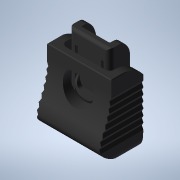
# Autodesk Inventor part: 6321.050_P9 1
Saved by Autodesk Inventor 2021 (Build 250183000, 183)
## iProperties
Created: 2025-05-05
Part Number: 6321.050_P9 1
Material: Generic
Catalog Web Link: www.cadenas.de
Description: AX Bediengehäuse für Tisch-TFT bis 24" - P9-Kompakt-Schaltschränke AX
Vendor: RITTAL
Document SubType Name: Modeling
Designer: psAdmin
Manufacturer: RITTAL
Mass: 3.67605 g
Surface Area: 33.3158 cm^2
Volume: 3.67605 cm^3
Density: 1 g/cm^3
Appearance: PSOLRGB-175-175-175
Category: PARTsolutions
Company: RITTAL
Title: 6321.050_P9 1
Author: Cadenas PARTsolutions
Comments: Kompakt-Schaltschränke AX
PSOL_IDENT_0: {$CADENAS_DATA/23d-libs/rittal/schaltschranksys/kompakt_schaltschr/parts_ae_2_0/bg_ax_fur_tisch_tft_
PSOL_IDENT_1: p9.prj},204 {VTYP=3D},{NB=6321.050_P9 1},{LINA=6321.050_P9 1},{NN=AX Bediengehäuse für Tisch-TFT bis
PSOL_IDENT_2: 24\" - P9},{DATE=28.04.2025 21:11:30},{GEOMDATE=11.04.2025 11:21:47},{VERSION=},{LINEID=40},{WBVAR=
PSOL_IDENT_3: },{WBNUMERIC=}  {NB=6321.050_P9 1},{LINA=6321.050_P9 1},{KT=DUMMY},{BEST=6321.050},{DETAIL=1},{B=650
PSOL_IDENT_4: },{H=450},{VER=1},{GEW=15,8},{CNSETIM80=EC002504},{CNSETIM90=EC002504},{CNSECLASS60=27-18-05-05},{CN
PSOL_IDENT_5: SECLASS80=27-18-05-05},{UNSPSC=31-26-15-02}
NB: 6321.050_P9 1
NN: AX Bediengehäuse für Tisch-TFT bis 24" - P9
NT: Kompakt-Schaltschränke AX
NBSYN: $BEST._P9 $DETAIL.
LINA: 6321.050_P9 1
CATALOG: Rittal
BEST: 6321.050
DETAIL: 1
B: 650
H: 450
VER: 1
GEW: 15,8
CNSETIM80: EC002504
CNSETIM90: EC002504
CNSECLASS60: 27-18-05-05
CNSECLASS80: 27-18-05-05
UNSPSC: 31-26-15-02
SUPPLIER: RITTAL
ARTICLENO: 6321.050_P9 1
BOMINFO: 6321.050_P9 1
CREATOR: CADENAS GmbH
Autodesk Inventor part; units mm, degrees
sketch "Sketch_1" plane through (0, 0, 0) normal (0, 0, 1) x (1, 0, 0)
  line L0 (-10.45, -19.2) -> (-10.45, -21.5)
  arc A0 (-10.45, -21.5) -> (-7.45, -24.5) centre (-7.45, -21.5) ccw
  line L1 (-7.45, -24.5) -> (-2.3229, -24.5)
  arc A1 (-2.3229, -24.5) -> (-1.6614, -24.25) centre (-2.3229, -23.5) ccw
  arc A2 (-1, -24) -> (-1.6614, -24.25) centre (-1, -25) ccw
  line L2 (-1, -24) -> (1, -24)
  arc A3 (1.6614, -24.25) -> (1, -24) centre (1, -25) ccw
  arc A4 (1.6614, -24.25) -> (2.3229, -24.5) centre (2.3229, -23.5) ccw
  line L3 (2.3229, -24.5) -> (7.45, -24.5)
  arc A5 (7.45, -24.5) -> (10.45, -21.5) centre (7.45, -21.5) ccw
  line L4 (10.45, -21.5) -> (10.45, -19.2)
  line L5 (10.45, -19.2) -> (9.95, -18.2)
  line L6 (9.95, -18.2) -> (10.45, -17.2)
  line L7 (10.45, -17.2) -> (9.95, -16.2)
  line L8 (9.95, -16.2) -> (10.45, -15.2)
  line L9 (10.45, -15.2) -> (9.95, -14.2)
  line L10 (9.95, -14.2) -> (10.45, -13.2)
  line L11 (10.45, -13.2) -> (9.95, -12.2)
  line L12 (9.95, -12.2) -> (10.45, -11.2)
  line L13 (10.45, -11.2) -> (9.95, -10.2)
  line L14 (9.95, -10.2) -> (10.45, -9.2)
  line L15 (10.45, -9.2) -> (9.95, -8.2)
  line L16 (9.95, -8.2) -> (10.45, -7.2)
  line L17 (10.45, -7.2) -> (9.95, -6.2)
  line L18 (9.95, -6.2) -> (10.45, -5.2)
  line L19 (10.45, -5.2) -> (10.45, -0.3)
  arc A6 (10.45, -0.3) -> (10.15, 0) centre (10.15, -0.3) ccw
  line L20 (10.15, 0) -> (-10.15, 0)
  arc A7 (-10.15, 0) -> (-10.45, -0.3) centre (-10.15, -0.3) ccw
  line L21 (-10.45, -0.3) -> (-10.45, -5.2)
  line L22 (-10.45, -5.2) -> (-9.95, -6.2)
  line L23 (-9.95, -6.2) -> (-10.45, -7.2)
  line L24 (-10.45, -7.2) -> (-9.95, -8.2)
  line L25 (-9.95, -8.2) -> (-10.45, -9.2)
  line L26 (-10.45, -9.2) -> (-9.95, -10.2)
  line L27 (-9.95, -10.2) -> (-10.45, -11.2)
  line L28 (-10.45, -11.2) -> (-9.95, -12.2)
  line L29 (-9.95, -12.2) -> (-10.45, -13.2)
  line L30 (-10.45, -13.2) -> (-9.95, -14.2)
  line L31 (-9.95, -14.2) -> (-10.45, -15.2)
  line L32 (-10.45, -15.2) -> (-9.95, -16.2)
  line L33 (-9.95, -16.2) -> (-10.45, -17.2)
  line L34 (-10.45, -17.2) -> (-9.95, -18.2)
  line L35 (-9.95, -18.2) -> (-10.45, -19.2)
  constraints: 72 end point, 16 point on circle, 8 centre point
extrude "Extrusion1" add sketch "Sketch_1" along normal blind 14
sketch "Sketch_2" plane through (0, 0, 0) normal (1, 0, 0) x (0, 1, 0)
  line L0 (-28, 20) -> (-28, -5)
  line L1 (-28, -5) -> (5, -5)
  line L2 (5, -5) -> (5, 20)
  line L3 (5, 20) -> (-28, 20)
  arc A0 (-18.0876, 13.9583) -> (-20.637, 12.9256) centre (-18.3613, 10.9708) ccw
  arc A1 (-20.637, 12.9256) -> (-24.5, 2.5) centre (-8.5, 2.5) ccw
  line L4 (-24.5, 2.5) -> (-24.5, 0.5657)
  arc A2 (-24.5, 0.5657) -> (-17, 0) centre (-17, 50) ccw
  line L5 (-17, 0) -> (-4, 0)
  arc A3 (-4, 0) -> (-3.4, 0.2) centre (-4, 1) ccw
  arc A4 (-3.4, 0.2) -> (0, 7) centre (-8.5, 7) ccw
  line L6 (0, 7) -> (0, 10.2)
  arc A5 (0, 10.2) -> (-0.3, 10.5) centre (-0.3, 10.2) ccw
  line L7 (-0.3, 10.5) -> (-3.744, 10.5)
  arc A6 (-14.614, 12.9868) -> (-3.744, 10.5) centre (-3.744, 35.5) ccw
  arc A7 (-14.614, 12.9868) -> (-18.0876, 13.9583) centre (-19, 4) ccw
  constraints: 16 end point, 16 point on circle, 8 centre point
extrude "Extrusion2" cut sketch "Sketch_2" along normal mid plane 22
sketch "Sketch_3" plane through (0, 0, 0) normal (0, 1, 0) x (-1, 0, 0)
  arc A0 (7.95, 1) -> (8.95, 0) centre (8.95, 1) ccw
  line L0 (7.95, 1) -> (7.95, 7)
  arc A1 (7.95, 7) -> (6.45, 8.5) centre (6.45, 7) ccw
  line L1 (6.45, 8.5) -> (-6.45, 8.5)
  arc A2 (-6.45, 8.5) -> (-7.95, 7) centre (-6.45, 7) ccw
  line L2 (-7.95, 7) -> (-7.95, 1)
  arc A3 (-8.95, 0) -> (-7.95, 1) centre (-8.95, 1) ccw
  line L3 (-8.95, 0) -> (8.95, 0)
  constraints: 8 end point, 8 point on circle, 4 centre point
extrude "Extrusion3" cut sketch "Sketch_3" against normal blind 17
sketch "Sketch_4" plane through (0, -17, 0) normal (0, 1, 0) x (1, 0, 0)
  arc A0 (-6.65, -5.7) -> (-5.15, -7.2) centre (-5.15, -5.7) ccw
  line L0 (-5.15, -7.2) -> (5.15, -7.2)
  arc A1 (5.15, -7.2) -> (6.65, -5.7) centre (5.15, -5.7) ccw
  line L1 (6.65, -5.7) -> (6.65, -1)
  arc A2 (6.65, -1) -> (5.65, 0) centre (5.65, -1) ccw
  line L2 (5.65, 0) -> (4.65, 0)
  line L3 (4.65, 0) -> (4.65, -4.9)
  arc A3 (4.35, -5.2) -> (4.65, -4.9) centre (4.35, -4.9) ccw
  line L4 (4.35, -5.2) -> (-4.35, -5.2)
  arc A4 (-4.65, -4.9) -> (-4.35, -5.2) centre (-4.35, -4.9) ccw
  line L5 (-4.65, -4.9) -> (-4.65, 0)
  line L6 (-4.65, 0) -> (-5.65, 0)
  arc A5 (-5.65, 0) -> (-6.65, -1) centre (-5.65, -1) ccw
  line L7 (-6.65, -1) -> (-6.65, -5.7)
  constraints: 16 end point, 12 point on circle, 6 centre point
extrude "Extrusion4" add sketch "Sketch_4" along normal blind 22
sketch "Sketch_5" plane through (0, 0, 0) normal (1, 0, 0) x (0, 1, 0)
  arc A0 (-17.5342, 10.9429) -> (-18.6481, 10.625) centre (-17.8675, 10) ccw
  arc A1 (-18.6481, 10.625) -> (-21.5, 2.5) centre (-8.5, 2.5) ccw
  line L0 (-21.5, 2.5) -> (-21.5, 0)
  line L1 (-21.5, 0) -> (0.812, 0)
  line L2 (0.812, 0) -> (0.812, 8.5)
  line L3 (0.812, 8.5) -> (-13.751, 8.5)
  arc A2 (-14.5155, 8.8554) -> (-13.751, 8.5) centre (-13.751, 9.5) ccw
  arc A3 (-14.5155, 8.8554) -> (-17.5342, 10.9429) centre (-19.867, 4.343) ccw
  constraints: 8 end point, 8 point on circle, 4 centre point
extrude "Extrusion5" cut sketch "Sketch_5" along normal mid plane 9.3
sketch "Sketch_6" plane through (0, 0, 0) normal (1, 0, 0) x (0, 1, 0)
  line L0 (7, 7.2) -> (4, 7.2)
  arc A0 (5, 6.2) -> (4, 7.2) centre (4, 6.2) ccw
  line L1 (5, 6.2) -> (5, 4)
  arc A1 (4.4748, 2.5371) -> (5, 4) centre (2.7, 4) ccw
  arc A2 (2.0035, 0.8591) -> (4.4748, 2.5371) centre (-0.17, 6.719) ccw
  arc A3 (-3, 0) -> (2.0035, 0.8591) centre (-3, 15) ccw
  line L2 (-3, 0) -> (-3, -0.8)
  line L3 (-3, -0.8) -> (7, -0.8)
  line L4 (7, -0.8) -> (7, 7.2)
  constraints: 10 end point, 8 point on circle, 4 centre point
extrude "Extrusion6" cut sketch "Sketch_6" along normal mid plane 14
sketch "Sketch_8" plane through (0, 0, 8.5) normal (0, 0, 1) x (1, 0, 0)
  arc A0 (-4.3301, -4.75) -> (4.3301, -4.75) centre (0, -7.25) ccw
  arc A1 (4.3301, -4.75) -> (2.5981, -3.75) centre (2.5981, -5.75) ccw
  line L0 (2.5981, -3.75) -> (-2.5981, -3.75)
  arc A2 (-2.5981, -3.75) -> (-4.3301, -4.75) centre (-2.5981, -5.75) ccw
  constraints: 6 point on circle, 3 centre point, 2 end point
extrude "Extrusion7" cut sketch "Sketch_8" along normal blind 5
sketch "Sketch_7" plane through (0, 0, 7.2) normal (0, 0, 1) x (1, 0, 0)
  arc A0 (-3.75, -7.888) -> (3.75, -7.888) centre (0, -7.888) ccw
  line L0 (3.75, -7.888) -> (3.75, 0.812)
  line L1 (3.75, 0.812) -> (-3.75, 0.812)
  line L2 (-3.75, 0.812) -> (-3.75, -7.888)
  constraints: 6 end point, 2 point on circle, 1 centre point
extrude "Extrusion8" add sketch "Sketch_7" against normal blind 2
sketch "Sketch_9" plane through (0, 0, 7.2) normal (0, 0, 1) x (1, 0, 0)
  circle A0 centre (0, -7.888) radius 3.75
  constraints: 1 centre point
extrude "Extrusion9" add sketch "Sketch_9" along normal blind 1.6
sketch "Sketch_10" plane through (0, 0, 0) normal (1, 0, 0) x (0, 1, 0)
  line L0 (-3.821, 8.8) -> (-11.638, 8.8)
  line L1 (-11.638, 8.8) -> (-11.638, 8.738)
  line L2 (-11.638, 8.738) -> (-11.178, 8.738)
  line L3 (-11.178, 8.738) -> (-9.2768, 8.4708)
  arc A0 (-7.9221, 8.0796) -> (-9.2768, 8.4708) centre (-9.9727, 3.5195) ccw
  arc A1 (-7.9221, 8.0796) -> (-3.821, 7.2) centre (-3.821, 17.2) ccw
  line L4 (-3.821, 7.2) -> (-3.821, 8.8)
  constraints: 10 end point, 4 point on circle, 2 centre point
extrude "Extrusion10" cut sketch "Sketch_10" along normal mid plane 7.5
sketch "Sketch_11" plane through (0, 0, 8.5) normal (0, 0, 1) x (1, 0, 0)
  circle A0 centre (0, -7.25) radius 6
  arc A1 (-4.3301, -4.75) -> (4.3301, -4.75) centre (0, -7.25) ccw
  arc A2 (4.3301, -4.75) -> (2.5981, -3.75) centre (2.5981, -5.75) ccw
  line L0 (2.5981, -3.75) -> (-2.5981, -3.75)
  arc A3 (-2.5981, -3.75) -> (-4.3301, -4.75) centre (-2.5981, -5.75) ccw
  constraints: 6 point on circle, 4 centre point, 2 end point
extrude "Extrusion11" add sketch "Sketch_11" along normal blind 1
sketch "Sketch_12" plane through (0, 0, 7.2) normal (0, 0, 1) x (1, 0, 0)
  arc A0 (-2.491, -5.6198) -> (-2.491, -9.3102) centre (0, -7.465) ccw
  arc A1 (-2.491, -9.3102) -> (-1.6875, -9.715) centre (-1.6875, -8.715) ccw
  line L0 (-1.6875, -9.715) -> (1.6875, -9.715)
  arc A2 (1.6875, -9.715) -> (2.491, -9.3102) centre (1.6875, -8.715) ccw
  arc A3 (2.491, -9.3102) -> (2.491, -5.6198) centre (0, -7.465) ccw
  arc A4 (2.491, -5.6198) -> (1.6875, -5.215) centre (1.6875, -6.215) ccw
  line L1 (1.6875, -5.215) -> (-1.6875, -5.215)
  arc A5 (-1.6875, -5.215) -> (-2.491, -5.6198) centre (-1.6875, -6.215) ccw
  constraints: 12 point on circle, 6 centre point, 4 end point
extrude "Extrusion12" cut sketch "Sketch_12" along normal blind 1.6
ref_plane "P9_XY" through (0, -7.5, 8.45) normal (0, 0, 1) x (1, 0, 0)
ref_plane "P9_YZ" through (0, -7.5, 8.45) normal (1, 0, 0) x (0, 1, 0)
ref_plane "P9_ZX" through (0, -7.5, 8.45) normal (0, 1, 0) x (0, 0, 1)
body "Solid1"
